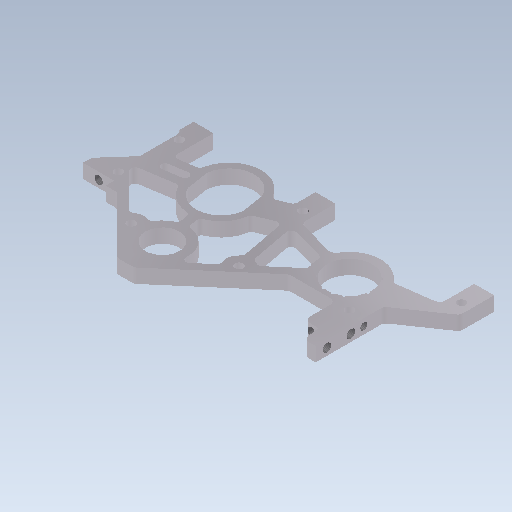
# Autodesk Inventor part: Bulkhead_RR
Saved by Autodesk Inventor 2020 (Build 240168000, 168)
## iProperties
Created: 2007-02-07
Part Number: Bulkhead_RR
Material: Steel
Document SubType Name: Modeling
Designer: Garin
Density: 7.85 g/cm^3
Appearance: Aluminum (Polished)
Mass: 64.7451 g
Surface Area: 78.6196 cm^2
Volume: 8.24779 cm^3
Translation Standard: STEP AP214IS
File Name: D:\My Workspace\Inventor\R11_XR_RCCar\Workspace\Parts\Bulkhead_RR.stp
Preprocessor: Autodesk Inventor 11
Postprocessor: Build: 535a, Release: 11 SP2 - Date: Mon 08/21/2006
Sent Units: MILLIMETERS
Uncertainty: 0.01
Author: Garin
Autodesk Inventor part; units mm, degrees
note: some values were not read from the file. Chosen so that the rebuilt part matches the saved one: direction of "Hole13"; direction of "Hole12"; direction of "Hole11"; direction of "Hole10"; direction of "Hole9"; direction of "Hole8"; direction of "Hole7"; direction of "Hole6"; direction of "Hole5"; direction of "Hole4"; direction of "Hole23".
ref_plane "YZ Plane" through (0, 0, 0) normal (1, 0, 0) x (0, 1, 0)
ref_plane "XZ Plane" through (0, 0, 0) normal (0, 1, 0) x (-1, 0, 0)
ref_plane "Work Plane1" through (0, 21.5, 0) normal (0, 1, 0) x (-1, 0, 0)
sketch "Sketch1" plane through (0, 21.5, 0) normal (0, 1, 0) x (-1, 0, 0)
  line L0 (-214.5, 0) -> (-221.5, 0)
  line L1 (-257.5, 0) -> (-257.5, 7.4004)
  line L2 (-257.5, 0) -> (-264.5, 0)
  line L3 (-264.5, 0) -> (-264.5, 12)
  line L4 (-264.5, 12) -> (-279.253, 16)
  arc A0 (-298.7195, 14) -> (-279.253, 16) centre (-289.5, 20) ccw
  line L5 (-313.5, 12) -> (-298.7195, 14)
  line L6 (-313.5, 0) -> (-313.5, 12)
  line L7 (-313.5, 0) -> (-320.5, 0)
  line L8 (-320.5, 12) -> (-320.5, 0)
  line L9 (-320.5, 12) -> (-304.5, 23)
  line L10 (-304.5, 47) -> (-304.5, 23)
  line L11 (-304.5, 47) -> (-300.5, 47)
  line L12 (-300.5, 47) -> (-299.5, 41)
  line L13 (-294.5, 41) -> (-294.5, 31)
  line L14 (-294.5, 31) -> (-276.5, 31)
  line L15 (-299.5, 41) -> (-294.5, 41)
  line L16 (-221.5, 14.4754) -> (-221.5, 0)
  line L17 (-214.5, 0) -> (-214.5, 5)
  line L18 (-229.9363, 13.1775) -> (-221.5, 14.4754)
  arc A1 (-251.6805, 9.8322) -> (-229.9363, 13.1775) centre (-241.2233, 14.2015) ccw
  line L19 (-257.5, 7.4004) -> (-251.6805, 9.8322)
  line L20 (-276.5, 31) -> (-248.5, 55)
  line L21 (-242.5, 55) -> (-248.5, 55)
  line L22 (-242.5, 55) -> (-222.5, 35)
  line L23 (-207.5, 35) -> (-222.5, 35)
  line L24 (-207.5, 35) -> (-207.5, 29)
  line L25 (-207.5, 29) -> (-215.5, 20)
  line L26 (-215.5, 20) -> (-215.5, 6.7321)
  arc A2 (-215.5, 6.7321) -> (-214.5, 5) centre (-213.5, 6.7321) ccw
  constraints: 54 end point, 10 vertical, 8 horizontal, 6 equal length, 6 point on circle, 3 centre point
extrude "Extrude8" add sketch "Sketch1" against normal blind 5 draft 0
fillet "Fillet1" radius 2 1 edges at (294.5, 19, 41)
fillet "Fillet1" radius 2 1 edges at (300.5, 19, 47)
fillet "Fillet1" radius 2 1 edges at (294.5, 19, 31)
fillet "Fillet1" radius 2 1 edges at (276.5, 19, 31)
fillet "Fillet1" radius 2 1 edges at (248.5, 19, 55)
fillet "Fillet1" radius 2 1 edges at (242.5, 19, 55)
fillet "Fillet1" radius 2 1 edges at (222.5, 19, 35)
fillet "Fillet1" radius 2 1 edges at (207.5, 19, 29)
fillet "Fillet1" radius 2 1 edges at (215.5, 19, 20)
fillet "Fillet1" radius 1.5 1 edges at (221.5, 19, 14.4754)
fillet "Fillet1" radius 1.5 1 edges at (229.9363, 19, 13.1775)
fillet "Fillet1" radius 1.5 1 edges at (251.6805, 19, 9.8322)
fillet "Fillet1" radius 1.5 1 edges at (257.5, 19, 7.4004)
fillet "Fillet1" radius 2 1 edges at (264.5, 19, 12)
fillet "Fillet1" radius 2 1 edges at (279.253, 19, 16)
fillet "Fillet1" radius 2 1 edges at (298.7195, 19, 14)
fillet "Fillet1" radius 2 1 edges at (313.5, 19, 12)
fillet "Fillet1" radius 2 1 edges at (320.5, 19, 12)
fillet "Fillet1" radius 2 1 edges at (304.5, 19, 23)
sketch "Sketch2" plane through (207.5, 16.5, 35) normal (0, 0, 1) x (1, 0, 0)
  line L0 (11, 0) -> (0, 0)
  line L1 (11, 5) -> (0, 5)
  line L2 (0, 5) -> (0, 0)
  line L3 (11, 5) -> (11, 0)
  constraints: 8 end point, 2 horizontal, 2 vertical
extrude "Extrude7" cut sketch "Sketch2" against normal blind 3 draft 0
sketch "Sketch3" plane through (0, 21.5, 0) normal (0, 1, 0) x (-1, 0, 0)
  line L0 (-233.6945, 21.1644) -> (-232.4567, 13.1183)
  arc A0 (-233.6945, 21.1644) -> (-250.4968, 18.5794) centre (-241.7302, 17.4961) ccw
  line L1 (-249.259, 10.5333) -> (-250.4968, 18.5794)
  arc A1 (-249.259, 10.5333) -> (-232.4567, 13.1183) centre (-241.2233, 14.2015) ccw
  constraints: 4 end point, 4 point on circle, 2 centre point, 2 parallel
extrude "Extrude6" cut sketch "Sketch3" against normal blind 5 draft 0
sketch "Sketch4" plane through (0, 21.5, 0) normal (0, 1, 0) x (-1, 0, 0)
  arc A0 (-294.489, 26.2538) -> (-295.9654, 24.7115) centre (-289.5, 20) ccw
  arc A1 (-295.9654, 24.7115) -> (-296.5025, 23.8685) centre (-296.2471, 24.2984) ccw
  arc A2 (-296.5025, 23.8685) -> (-297.2763, 21.8786) centre (-289.5, 20) ccw
  arc A3 (-297.2763, 21.8786) -> (-297.4499, 20.8943) centre (-297.3785, 21.3892) ccw
  arc A4 (-297.4499, 20.8943) -> (-295.9376, 15.2506) centre (-289.5, 20) ccw
  arc A5 (-295.9376, 15.2506) -> (-295.2951, 14.4849) centre (-295.6284, 14.8577) ccw
  arc A6 (-295.2951, 14.4849) -> (-283.0624, 24.7494) centre (-289.5, 20) ccw
  arc A7 (-283.0624, 24.7494) -> (-283.7049, 25.5151) centre (-283.3716, 25.1423) ccw
  arc A8 (-283.7049, 25.5151) -> (-287.6214, 27.7763) centre (-289.5, 20) ccw
  arc A9 (-287.6214, 27.7763) -> (-288.6057, 27.9499) centre (-288.1108, 27.8785) ccw
  arc A10 (-288.6057, 27.9499) -> (-290.7402, 27.9033) centre (-289.5, 20) ccw
  arc A11 (-290.7402, 27.9033) -> (-291.716, 27.6869) centre (-291.2315, 27.8104) ccw
  arc A12 (-291.716, 27.6869) -> (-293.6703, 26.8271) centre (-289.5, 20) ccw
  arc A13 (-293.6703, 26.8271) -> (-294.489, 26.2538) centre (-294.0886, 26.5532) ccw
  constraints: 28 point on circle, 14 centre point
extrude "Extrude5" cut sketch "Sketch4" against normal blind 5 draft 0
sketch "Sketch5" plane through (0, 21.5, 0) normal (0, 1, 0) x (-1, 0, 0)
  line L0 (-261.9639, 39.5083) -> (-256.9553, 43.8014)
  arc A0 (-261.9639, 39.5083) -> (-262.3658, 37.7771) centre (-260.9877, 38.3694) ccw
  arc A1 (-263.5714, 32.5833) -> (-262.3658, 37.7771) centre (-266.5, 36) ccw
  arc A2 (-263.5714, 32.5833) -> (-264.0696, 31.1685) centre (-262.5953, 31.4445) ccw
  line L1 (-261.4135, 16.9774) -> (-264.0696, 31.1685)
  arc A3 (-261.4135, 16.9774) -> (-259.3608, 15.8693) centre (-259.9391, 17.2534) ccw
  line L2 (-253.8164, 18.1862) -> (-259.3608, 15.8693)
  arc A4 (-253.8164, 18.1862) -> (-252.9145, 19.3278) centre (-254.3948, 19.5702) ccw
  arc A5 (-246.0243, 27.9844) -> (-252.9145, 19.3278) centre (-241.7302, 17.4961) ccw
  arc A6 (-246.0243, 27.9844) -> (-245.1101, 29.6007) centre (-246.5926, 29.3726) ccw
  line L3 (-245.4525, 31.8266) -> (-245.1101, 29.6007)
  arc A7 (-245.4525, 31.8266) -> (-246.7301, 33.0845) centre (-246.9351, 31.5985) ccw
  arc A8 (-254.4821, 42.5679) -> (-246.7301, 33.0845) centre (-245.5, 42) ccw
  arc A9 (-254.4821, 42.5679) -> (-256.9553, 43.8014) centre (-255.9791, 42.6625) ccw
  constraints: 20 point on circle, 10 centre point, 8 end point
extrude "Extrude4" cut sketch "Sketch5" against normal blind 5 draft 0
sketch "Sketch6" plane through (0, 21.5, 0) normal (0, 1, 0) x (-1, 0, 0)
  arc A0 (-241.647, 33.8665) -> (-242.4874, 32.2828) centre (-241.0048, 32.5109) ccw
  line L0 (-242.1449, 30.0569) -> (-242.4874, 32.2828)
  arc A1 (-242.1449, 30.0569) -> (-240.7872, 28.7902) centre (-240.6624, 30.285) ccw
  arc A2 (-231.7219, 22.814) -> (-240.7872, 28.7902) centre (-241.7302, 17.4961) ccw
  arc A3 (-231.7219, 22.814) -> (-230.1692, 22.0353) centre (-230.3973, 23.5178) ccw
  line L1 (-218.8891, 23.7707) -> (-230.1692, 22.0353)
  arc A4 (-218.8891, 23.7707) -> (-218.0565, 26.3139) centre (-219.1172, 25.2532) ccw
  line L2 (-229.9339, 38.1912) -> (-218.0565, 26.3139)
  arc A5 (-229.9339, 38.1912) -> (-231.8709, 38.3479) centre (-230.9945, 37.1305) ccw
  arc A6 (-236.0938, 37.7917) -> (-231.8709, 38.3479) centre (-234.5, 42) ccw
  arc A7 (-236.0938, 37.7917) -> (-237.8929, 37.1905) centre (-236.625, 36.3889) ccw
  arc A8 (-241.647, 33.8665) -> (-237.8929, 37.1905) centre (-245.5, 42) ccw
  constraints: 18 point on circle, 9 centre point, 6 end point, 1 perpendicular
extrude "Extrude3" cut sketch "Sketch6" against normal blind 5 draft 0
sketch "Sketch7" plane through (0, 21.5, 0) normal (0, 1, 0) x (-1, 0, 0)
  line L0 (-222.968, 17.2848) -> (-228.9245, 16.3684)
  arc A0 (-222.968, 17.2848) -> (-221.6962, 18.7859) centre (-223.1961, 18.7674) ccw
  arc A1 (-221.6962, 18.7859) -> (-223.4068, 20.0403) centre (-223.1787, 18.5578) ccw
  line L1 (-229.3342, 19.1284) -> (-223.4068, 20.0403)
  arc A2 (-229.3342, 19.1284) -> (-230.5887, 17.4178) centre (-229.1061, 17.6459) ccw
  arc A3 (-230.5887, 17.4178) -> (-228.9245, 16.3684) centre (-229.1526, 17.851) ccw
  constraints: 8 point on circle, 4 centre point, 4 end point, 1 parallel
extrude "Extrude2" cut sketch "Sketch7" against normal blind 5 draft 0
sketch "Sketch8" plane through (0, 21.5, 0) normal (0, 1, 0) x (-1, 0, 0)
  arc A0 (-268.8885, 32.1862) -> (-267.9946, 31.7555) centre (-266.5, 36) ccw
  arc A1 (-266.4018, 15.624) -> (-264.5349, 17.3477) centre (-266.0093, 17.0717) ccw
  line L0 (-267.0184, 30.6166) -> (-264.5349, 17.3477)
  arc A2 (-267.0184, 30.6166) -> (-267.9946, 31.7555) centre (-268.4928, 30.3406) ccw
  arc A3 (-268.8885, 32.1862) -> (-270.6608, 32.0538) centre (-269.6846, 30.9149) ccw
  line L1 (-278.6549, 25.2017) -> (-270.6608, 32.0538)
  arc A4 (-278.6549, 25.2017) -> (-279.0972, 23.5753) centre (-277.6787, 24.0628) ccw
  arc A5 (-278.5001, 20.0454) -> (-279.0972, 23.5753) centre (-289.5, 20) ccw
  arc A6 (-278.5001, 20.0454) -> (-277.3926, 18.6039) centre (-277.0001, 20.0516) ccw
  line L2 (-266.4018, 15.624) -> (-277.3926, 18.6039)
  constraints: 14 point on circle, 7 centre point, 6 end point
extrude "Extrude1" cut sketch "Sketch8" against normal blind 5 draft 0
hole "Hole15" at (213, 19, 32) direction (0, 0, -1) diameter 3 depth 6 tip angle 118
hole "Hole14" at (297, 19, 41) direction (0, 0, -1) diameter 3 depth 4 tip angle 118
hole "Hole13" at (304.5, 19, 43) direction (-1, 0, 0) diameter 3 end up to surface
hole "Hole12" at (217.5, 16.5, 8) direction (0, 1, 0) diameter 3 depth 5
hole "Hole11" at (234.5, 16.5, 42) direction (0, 1, 0) diameter 3 depth 5
hole "Hole10" at (261, 16.5, 8) direction (0, 1, 0) diameter 3 depth 5
hole "Hole9" at (294.5, 19, 34.5) direction (1, 0, 0) diameter 3 depth 10
sketch "Sketch16" plane through (0, 16.5, 0) normal (0, -1, 0) x (1, 0, 0)
  point P0 (299.5, 30)
hole "Hole8" at (299.5, 16.5, 30) direction (0, 1, 0) diameter 3 depth 5
sketch "Sketch15" plane through (294.5, 21.5, 33) normal (-1, 0, 0) x (0, 0, 1)
  point P0 (1.5, -2.5)
hole "Hole7" at (266.5, 16.5, 36) direction (0, 1, 0) diameter 3 depth 5
sketch "Sketch14" plane through (0, 16.5, 0) normal (0, -1, 0) x (1, 0, 0)
  point P0 (261, 8)
hole "Hole6" at (216.5, 16.5, 28.5) direction (0, 1, 0) diameter 3 depth 5
sketch "Sketch13" plane through (0, 16.5, 0) normal (0, -1, 0) x (1, 0, 0)
  point P0 (234.5, 42)
hole "Hole5" at (245.5, 16.5, 42) direction (0, 1, 0) diameter 12 depth 5
sketch "Sketch12" plane through (0, 16.5, 0) normal (0, -1, 0) x (1, 0, 0)
  point P0 (217.5, 8)
hole "Hole4" at (317, 16.5, 8) direction (0, 1, 0) diameter 3 depth 5
sketch "Sketch11" plane through (304.5, 16.5, 47) normal (1, 0, 0) x (0, 0, -1)
  point P0 (4, 2.5)
hole "Hole3" at (261, 19, 0) direction (0, 0, 1) diameter 3 depth 5
sketch "Sketch10" plane through (299.5, 16.5, 41) normal (0, 0, 1) x (1, 0, 0)
  point P0 (-2.5, 2.5)
hole "Hole2" at (218, 19, 0) direction (0, 0, 1) diameter 3 depth 5
sketch "Sketch9" plane through (207.5, 16.5, 32) normal (0, 0, 1) x (1, 0, 0)
  point P0 (5.5, 2.5)
hole "Hole1" at (317, 19, 0) direction (0, 0, 1) diameter 3 depth 5
thread "Thread1" size "M3x0.5" class "6H" standard "ISO Metric profile" full length
thread "Thread2" size "M3x0.5" class "6H" standard "ISO Metric profile" full length
thread "Thread3" size "M3x0.5" class "6H" standard "ISO Metric profile" full length
thread "Thread4" size "M3x0.5" class "6H" standard "ISO Metric profile" full length
thread "Thread5" size "M3x0.5" class "6H" standard "ISO Metric profile" full length
thread "Thread6" size "M3x0.5" class "6H" standard "ANSI Metric M Profile" full length
thread "Thread7" size "M3x0.5" class "6H" standard "ISO Metric profile" full length
sketch "Sketch26" plane through (304.5, 16.5, 47) normal (1, 0, 0) x (0, 0, -1)
  circle A0 centre (12.5, 2.5) radius 1.5 projected
  line L0 (0, 5) -> (0, 0) projected
  point P0 (47, -16.5)
  point P1 (17, 2.5)
  dimension "d165" = 17
  constraints: 1 horizontal alignment
  measures "d165" distance from line of L0 point (17, 2.5)
hole "Hole23" at (304.5, 19, 30) direction (-1, 0, 0) diameter 2.459 end up to surface thread size "M3x0.5" class "6H" standard "ANSI Metric M Profile"
sketch "Sketch27" plane through (0, 16.5, 0) normal (0, -1, 0) x (1, 0, 0)
  line L0 (249.0617, 54.5185) -> (275.9383, 31.4815) projected
  line L1 (218.5, 35) -> (218.5, 32) projected
  line L2 (277.9462, 29.7604) -> (294.5, 29.7604)
  line L3 (277.9462, 29.7604) -> (275.9383, 31.4815)
  line L4 (294.5, 29.7604) -> (294.5, 33)
  line L5 (275.9383, 31.4815) -> (294.5, 33)
  point P0 (0, 0)
  dimension "d145" = 3
  dimension "d146" = 4
  constraints: 8 end point, 2 perpendicular, 1 collinear
extrude "Extrusion11" cut sketch "Sketch27" against normal up to next
fillet "Fillet2" radius 2 2 edges at (277.9462, 19, 29.7604) (294.5, 19, 29.7604)
sketch "Sketch17" plane through (0, 16.5, 0) normal (0, -1, 0) x (1, 0, 0)
  point P0 (266.5, 36)
sketch "Sketch18" plane through (0, 16.5, 0) normal (0, -1, 0) x (1, 0, 0)
  point P0 (216.5, 28.5)
sketch "Sketch19" plane through (0, 16.5, 0) normal (0, -1, 0) x (1, 0, 0)
  point P0 (245.5, 42)
sketch "Sketch20" plane through (0, 16.5, 0) normal (0, -1, 0) x (1, 0, 0)
  point P0 (317, 8)
sketch "Sketch21" plane through (0, 0, 0) normal (0, 0, 1) x (1, 0, 0)
  point P0 (261, 19)
sketch "Sketch22" plane through (0, 0, 0) normal (0, 0, 1) x (1, 0, 0)
  point P0 (218, 19)
sketch "Sketch23" plane through (0, 0, 0) normal (0, 0, 1) x (1, 0, 0)
  point P0 (317, 19)
body "Solid1"
